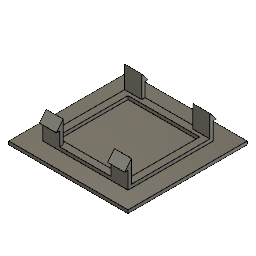
faceplate (Autodesk Fusion 360 design; units mm, degrees)
Autodesk Fusion 360 part; units mm, degrees
sketch "Sketch1" plane through (0, 0, 0) normal (0, 1, 0) x (1, 0, 0)
  line L0 (5.08, -7.62) -> (93.98, -7.62)
  line L1 (93.98, -7.62) -> (93.98, -96.52)
  line L2 (93.98, -96.52) -> (5.08, -96.52)
  line L3 (5.08, -96.52) -> (5.08, -7.62)
  dimension "d1" = 88.9
  dimension "d2" = 88.9
  constraint horizontal L0
  constraint vertical L1
  constraint horizontal L2
  constraint vertical L3
  measures "d1" distance of L0.start L0.end
  measures "d2" distance of L0.start L2.end
extrude "Extrude1" add sketch "Sketch1" along normal blind 2.54
sketch "Sketch2" plane through (0, 2.54, 0) normal (0, 1, 0) x (-1, 0, 0)
  line L0 (-5.08, 96.52) -> (-93.98, 96.52)
  line L1 (-93.98, 96.52) -> (-93.98, 7.62)
  line L2 (-93.98, 7.62) -> (-5.08, 7.62)
  line L3 (-5.08, 7.62) -> (-5.08, 96.52)
  line L4 (-17.78, 20.32) -> (-81.28, 20.32)
  line L5 (-81.28, 20.32) -> (-81.28, 83.82)
  line L6 (-81.28, 83.82) -> (-17.78, 83.82)
  line L7 (-17.78, 83.82) -> (-17.78, 20.32)
  dimension "d5" = 63.5
  dimension "d6" = 63.5
  dimension "d7" = 12.7
  dimension "d8" = 12.7
  constraint horizontal L4
  constraint vertical L5
  constraint horizontal L6
  constraint vertical L7
  measures "d5" distance of L4.start L4.end
  measures "d6" distance of L4.start L6.end
  measures "d7" distance of L2 L4
  measures "d8" distance of L3 L7
extrude "Extrude2" add sketch "Sketch2" along normal blind 2.54 contours L4 L5 L6 L7
sketch "Sketch3" plane through (0, 5.08, 0) normal (0, 1, 0) x (-1, 0, 0)
  line L0 (-17.78, 83.82) -> (-81.28, 83.82)
  line L1 (-81.28, 83.82) -> (-81.28, 20.32)
  line L2 (-81.28, 20.32) -> (-17.78, 20.32)
  line L3 (-17.78, 20.32) -> (-17.78, 83.82)
  line L4 (-17.78, 20.32) -> (-30.48, 20.32)
  line L5 (-30.48, 20.32) -> (-30.48, 22.86)
  line L6 (-30.48, 22.86) -> (-17.78, 22.86)
  line L7 (-17.78, 22.86) -> (-17.78, 20.32)
  line L8 (-81.28, 20.32) -> (-68.58, 20.32)
  line L9 (-68.58, 20.32) -> (-68.58, 22.86)
  line L10 (-68.58, 22.86) -> (-81.28, 22.86)
  line L11 (-81.28, 22.86) -> (-81.28, 20.32)
  line L12 (-17.78, 83.82) -> (-30.48, 83.82)
  line L13 (-30.48, 83.82) -> (-30.48, 81.28)
  line L14 (-30.48, 81.28) -> (-17.78, 81.28)
  line L15 (-17.78, 81.28) -> (-17.78, 83.82)
  line L16 (-81.28, 83.82) -> (-68.58, 83.82)
  line L17 (-68.58, 83.82) -> (-68.58, 81.28)
  line L18 (-68.58, 81.28) -> (-81.28, 81.28)
  line L19 (-81.28, 81.28) -> (-81.28, 83.82)
  constraint horizontal L4
  constraint vertical L5
  constraint horizontal L6
  constraint vertical L7
  constraint coincident L2.end L3.start
  constraint horizontal L8
  constraint vertical L9
  constraint horizontal L10
  constraint vertical L11
  constraint coincident L1.end L2.start
  constraint horizontal L12
  constraint vertical L13
  constraint horizontal L14
  constraint vertical L15
  constraint coincident L0.start L3.end
  constraint horizontal L16
  constraint vertical L17
  constraint horizontal L18
  constraint vertical L19
  constraint coincident L0.end L1.start
extrude "Extrude3" add sketch "Sketch3" along normal blind 10.31 contours L0 L3 L12 L13 L14 L15 | L0 L1 L16 L17 L18 L19 | L2 L3 L4 L5 L6 L7 | L1 L2 L8 L9 L10 L11
sketch "Sketch4" plane through (0, 15.39, 0) normal (0, 1, 0) x (-1, 0, 0)
  line L0 (-81.28, 81.28) -> (-68.58, 81.28)
  line L1 (-68.58, 81.28) -> (-68.58, 83.82)
  line L2 (-68.58, 83.82) -> (-81.28, 83.82)
  line L3 (-81.28, 83.82) -> (-81.28, 81.28)
  line L4 (-30.48, 81.28) -> (-17.78, 81.28)
  line L5 (-17.78, 81.28) -> (-17.78, 86.36)
  line L6 (-17.78, 86.36) -> (-30.48, 86.36)
  line L7 (-30.48, 86.36) -> (-30.48, 81.28)
  line L8 (-17.78, 22.86) -> (-30.48, 22.86)
  line L9 (-30.48, 22.86) -> (-30.48, 17.78)
  line L10 (-30.48, 17.78) -> (-17.78, 17.78)
  line L11 (-17.78, 17.78) -> (-17.78, 22.86)
  line L12 (-68.58, 22.86) -> (-81.28, 22.86)
  line L13 (-81.28, 22.86) -> (-81.28, 17.78)
  line L14 (-81.28, 17.78) -> (-68.58, 17.78)
  line L15 (-68.58, 17.78) -> (-68.58, 22.86)
  line L16 (-81.28, 81.28) -> (-68.58, 81.28)
  line L17 (-68.58, 81.28) -> (-68.58, 86.36)
  line L18 (-68.58, 86.36) -> (-81.28, 86.36)
  line L19 (-81.28, 86.36) -> (-81.28, 81.28)
  dimension "d17" = 5.08
  dimension "d18" = 5.08
  dimension "d19" = 5.08
  dimension "d20" = 5.08
  constraint horizontal L4
  constraint vertical L5
  constraint horizontal L6
  constraint vertical L7
  constraint horizontal L8
  constraint vertical L9
  constraint horizontal L10
  constraint vertical L11
  constraint horizontal L12
  constraint vertical L13
  constraint horizontal L14
  constraint vertical L15
  constraint horizontal L16
  constraint vertical L17
  constraint horizontal L18
  constraint vertical L19
  constraint coincident L0.start L3.end
  measures "d17" distance of L8.end L9.end
  measures "d18" distance of L12.end L13.end
  measures "d19" distance of L0.end L17.end
  measures "d20" distance of L4.end L5.end
extrude "Extrude4" add sketch "Sketch4" along normal blind 6.35
sketch "Sketch5" plane through (81.28, 0, 0) normal (1, 0, 0) x (0, 0, -1)
  line L0 (-83.82, 2.54) -> (-20.32, 2.54)
  line L1 (-20.32, 2.54) -> (-20.32, 15.39)
  line L2 (-20.32, 15.39) -> (-17.78, 15.39)
  line L3 (-17.78, 15.39) -> (-17.78, 21.74)
  line L4 (-17.78, 21.74) -> (-22.86, 21.74)
  line L5 (-22.86, 21.74) -> (-22.86, 5.08)
  line L6 (-22.86, 5.08) -> (-81.28, 5.08)
  line L7 (-81.28, 5.08) -> (-81.28, 21.74)
  line L8 (-81.28, 21.74) -> (-86.36, 21.74)
  line L9 (-86.36, 21.74) -> (-86.36, 15.39)
  line L10 (-86.36, 15.39) -> (-83.82, 15.39)
  line L11 (-83.82, 15.39) -> (-83.82, 2.54)
  line L12 (-86.36, 15.39) -> (-81.28, 21.74)
  line L13 (-86.36, 21.74) -> (-86.36, 15.39)
  line L14 (-81.28, 21.74) -> (-86.36, 21.74)
  line L15 (-22.86, 21.74) -> (-17.78, 15.39)
  line L16 (-17.78, 21.74) -> (-22.86, 21.74)
  constraint coincident L9.end L10.start
  constraint coincident L7.end L8.start
  constraint coincident L8.end L9.start
  constraint coincident L4.end L5.start
  constraint coincident L2.end L3.start
  constraint coincident L3.end L4.start
extrude "Extrude5" cut sketch "Sketch5" against normal blind 63.5 contours L8 L9 L12 L13 L14 | L3 L4 L15 L16
sketch "Sketch6" plane through (0, 5.08, 0) normal (0, 1, 0) x (-1, 0, 0)
  line L0 (-30.48, 81.28) -> (-30.48, 83.82)
  line L1 (-30.48, 83.82) -> (-68.58, 83.82)
  line L2 (-68.58, 83.82) -> (-68.58, 81.28)
  line L3 (-68.58, 81.28) -> (-81.28, 81.28)
  line L4 (-81.28, 81.28) -> (-81.28, 22.86)
  line L5 (-81.28, 22.86) -> (-68.58, 22.86)
  line L6 (-68.58, 22.86) -> (-68.58, 20.32)
  line L7 (-68.58, 20.32) -> (-30.48, 20.32)
  line L8 (-30.48, 20.32) -> (-30.48, 22.86)
  line L9 (-30.48, 22.86) -> (-17.78, 22.86)
  line L10 (-17.78, 22.86) -> (-17.78, 81.28)
  line L11 (-17.78, 81.28) -> (-30.48, 81.28)
  line L12 (-22.86, 78.74) -> (-76.2, 78.74)
  line L13 (-76.2, 78.74) -> (-76.2, 25.4)
  line L14 (-76.2, 25.4) -> (-22.86, 25.4)
  line L15 (-22.86, 25.4) -> (-22.86, 78.74)
  constraint horizontal L12
  constraint vertical L13
  constraint horizontal L14
  constraint vertical L15
extrude "Extrude6" cut sketch "Sketch6" against normal blind 2.54 contours L12 L13 L14 L15
equation "d11 = 0.4 in + 0.15 mm"
